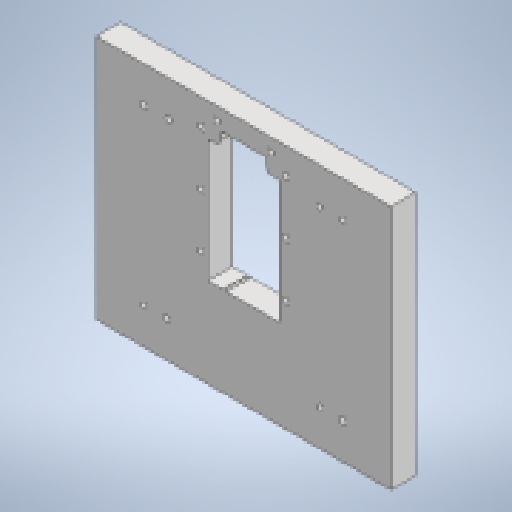
# Autodesk Inventor part: _body
Saved by Autodesk Inventor 2024.3 (Build 283343000, 343)
## iProperties
Created: 2024-09-06
Part Number: _body
Material: 일반
Document SubType Name: Modeling
Designer: gretc
Density: 1 g/cm^3
Appearance: 기본값
Author: gretc
Autodesk Inventor part; units mm, degrees
ref_plane "YZ Plane" through (0, 0, 0) normal (1, 0, 0) x (0, 1, 0)
ref_plane "XZ Plane" through (0, 0, 0) normal (0, 1, 0) x (-1, 0, 0)
ref_plane "XY Plane" through (0, 0, 0) normal (0, 0, 1) x (1, 0, 0)
ref_plane "작업 평면1" through (0, 0, 0) normal (0, 0, 1) x (1, 0, 0)
sketch "스케치1" plane through (0, 0, 0) normal (0, 0, 1) x (1, 0, 0)
  line L0 (-23.2, -18.48) -> (-93.2, -18.48) projected
  circle A0 centre (18.4, -3) radius 1.35 projected
  circle A1 centre (9.2, -3) radius 1.35 projected
  line L1 (0, 0) -> (27.6, 0) projected
  line L2 (0, 0) -> (0, -6) projected
  line L3 (0, -6) -> (27.6, -6) projected
  line L4 (27.6, 0) -> (27.6, -6) projected
  circle A2 centre (-62.8, -3) radius 1.35 projected
  circle A3 centre (-53.6, -3) radius 1.35 projected
  line L5 (-44.4, 0) -> (-72, 0) projected
  line L6 (-72, 0) -> (-72, -6) projected
  line L7 (-44.4, -6) -> (-72, -6) projected
  line L8 (-44.4, 0) -> (-44.4, -6) projected
  circle A4 centre (-62.8, 67.72) radius 1.35 projected
  circle A5 centre (-52.9755, 67.72) radius 1.35 projected
  line L9 (-44.4, 70.72) -> (-72, 70.72) projected
  line L10 (-72, 70.72) -> (-72, 64.72) projected
  line L11 (-44.4, 64.72) -> (-72, 64.72) projected
  line L12 (-44.4, 70.72) -> (-44.4, 64.72) projected
  circle A6 centre (18.4, 67.72) radius 1.35 projected
  circle A7 centre (8.5755, 67.72) radius 1.35 projected
  line L13 (0, 70.72) -> (27.6, 70.72) projected
  line L14 (0, 70.72) -> (0, 64.72) projected
  line L15 (0, 64.72) -> (27.6, 64.72) projected
  line L16 (27.6, 70.72) -> (27.6, 64.72) projected
  line L17 (0, 64.72) -> (-44.4, 64.72)
  line L18 (-44.4, 0) -> (-44.4, 64.72)
  line L19 (-22.2, 64.72) -> (-22.2, 32.36)
  line L20 (37.8, -17.64) -> (37.8, 82.36)
  line L21 (37.8, 82.36) -> (-82.2, 82.36)
  line L22 (-82.2, 82.36) -> (-82.2, -17.64)
  line L23 (-82.2, -17.64) -> (37.8, -17.64)
  line L24 (37.8, -17.64) -> (-82.2, 82.36) construction
  line L25 (37.8, 82.36) -> (-82.2, -17.64) construction
  dimension "d0" = 32.36
  dimension "d1" = 100
  dimension "d2" = 120
  constraints: 18 end point, 3 midpoint, 2 parallel, 2 perpendicular, 2 vertical, 1 collinear
  measures "d0" distance of L19.start L19.end
  measures "d1" distance of L20.start L20.end
  measures "d2" distance of L21.end L20.end
extrude "돌출1" add sketch "스케치1" along normal blind 10 contours L1 L4 L3 L2 | L8 L7 L6 L5 | L12 L11 L10 L9 | L13 L16 L15 L14 | L23 L22 L21 L20
sketch "스케치3" plane through (0, 0, 10) normal (0, 0, 1) x (1, 0, 0)
  arc A0 (-42.3, 27.1781) -> (-41.7808, 25.4912) centre (-39.3, 27.1781) ccw projected
  line L0 (-41.7808, 25.4912) -> (-37.7953, 19.6301) projected
  arc A1 (-37.7953, 19.6301) -> (-36.1414, 18.7547) centre (-36.1414, 20.7547) ccw projected
  line L1 (-35.2, 18.7547) -> (-36.1414, 18.7547) projected
  arc A2 (-36.7, 20.2547) -> (-35.2, 18.7547) centre (-35.2, 20.2547) ccw projected
  line L2 (-36.7, 73.2547) -> (-36.7, 20.2547) projected
  arc A3 (-35.7, 74.2547) -> (-36.7, 73.2547) centre (-35.7, 73.2547) ccw projected
  line L3 (-8.7, 74.2547) -> (-35.7, 74.2547) projected
  arc A4 (-7.7, 73.2547) -> (-8.7, 74.2547) centre (-8.7, 73.2547) ccw projected
  line L4 (-7.7, 20.2547) -> (-7.7, 73.2547) projected
  arc A5 (-9.2, 18.7547) -> (-7.7, 20.2547) centre (-9.2, 20.2547) ccw projected
  line L5 (-8.2586, 18.7547) -> (-9.2, 18.7547) projected
  arc A6 (-8.2586, 18.7547) -> (-6.6047, 19.6301) centre (-8.2586, 20.7547) ccw projected
  line L6 (-6.6047, 19.6301) -> (-2.6192, 25.4912) projected
  arc A7 (-2.6192, 25.4912) -> (-2.1, 27.1781) centre (-5.1, 27.1781) ccw projected
  line L7 (-2.1, 27.1781) -> (-2.1, 71.4314) projected
  arc A8 (-2.1, 71.4314) -> (-2.6192, 73.1183) centre (-5.1, 71.4314) ccw projected
  line L8 (-2.6192, 73.1183) -> (-6.3071, 78.5417) projected
  arc A9 (-6.3071, 78.5417) -> (-8.7879, 79.8547) centre (-8.7879, 76.8547) ccw projected
  line L9 (-8.7879, 79.8547) -> (-35.6121, 79.8547) projected
  arc A10 (-35.6121, 79.8547) -> (-38.0929, 78.5417) centre (-35.6121, 76.8547) ccw projected
  line L10 (-38.0929, 78.5417) -> (-41.7808, 73.1183) projected
  arc A11 (-41.7808, 73.1183) -> (-42.3, 71.4314) centre (-39.3, 71.4314) ccw projected
  line L11 (-42.3, 71.4314) -> (-42.3, 27.1781) projected
  circle A12 centre (-4.9, 27.7547) radius 1.35 projected
  circle A13 centre (-4.9, 49.7547) radius 1.35 projected
  circle A14 centre (-11.2, 77.0547) radius 1.35 projected
  circle A15 centre (-39.5, 27.7547) radius 1.35 projected
  circle A16 centre (-39.5, 49.7547) radius 1.35 projected
  circle A17 centre (-33.2, 77.0547) radius 1.35 projected
  circle A18 centre (-4.9, 71.7547) radius 1.35 projected
  circle A19 centre (-39.5, 71.7547) radius 1.35 projected
  point P0 (0, 0)
extrude "돌출2" cut sketch "스케치3" against normal blind 10 contours A12 | A13 | A14 | A15 | A16 | A17 | A18 | A19
sketch "스케치4" plane through (0, 0, 10) normal (0, 0, 1) x (1, 0, 0)
  circle A0 centre (-22.2, 31.7547) radius 7.5 projected
  circle A1 centre (-22.2, 31.7547) radius 7.5 projected
  point P0 (0, 0)
extrude "돌출3" cut sketch "스케치4" against normal blind 10
sketch "스케치5" plane through (0, 0, 10) normal (0, 0, 1) x (1, 0, 0)
  arc A0 (-42.3, 27.1781) -> (-41.7808, 25.4912) centre (-39.3, 27.1781) ccw projected
  line L0 (-42.3, 71.4314) -> (-42.3, 27.1781) projected
  arc A1 (-41.7808, 73.1183) -> (-42.3, 71.4314) centre (-39.3, 71.4314) ccw projected
  line L1 (-38.0929, 78.5417) -> (-41.7808, 73.1183) projected
  arc A2 (-35.6121, 79.8547) -> (-38.0929, 78.5417) centre (-35.6121, 76.8547) ccw projected
  line L2 (-8.7879, 79.8547) -> (-35.6121, 79.8547) projected
  arc A3 (-6.3071, 78.5417) -> (-8.7879, 79.8547) centre (-8.7879, 76.8547) ccw projected
  line L3 (-2.6192, 73.1183) -> (-6.3071, 78.5417) projected
  arc A4 (-2.1, 71.4314) -> (-2.6192, 73.1183) centre (-5.1, 71.4314) ccw projected
  line L4 (-2.1, 27.1781) -> (-2.1, 71.4314) projected
  arc A5 (-2.6192, 25.4912) -> (-2.1, 27.1781) centre (-5.1, 27.1781) ccw projected
  line L5 (-6.6047, 19.6301) -> (-2.6192, 25.4912) projected
  arc A6 (-8.2586, 18.7547) -> (-6.6047, 19.6301) centre (-8.2586, 20.7547) ccw projected
  line L6 (-14.55, 18.7547) -> (-8.2586, 18.7547) projected
  arc A7 (-14.55, 18.7547) -> (-13.05, 20.2547) centre (-14.55, 20.2547) ccw projected
  line L7 (-13.05, 20.2547) -> (-13.05, 21.7547) projected
  arc A8 (-10.7, 24.1047) -> (-13.05, 21.7547) centre (-10.7, 21.7547) ccw projected
  line L8 (-10.7, 24.1047) -> (-8.7, 24.1047) projected
  arc A9 (-8.7, 24.1047) -> (-7.7, 25.1047) centre (-8.7, 25.1047) ccw projected
  line L9 (-7.7, 25.1047) -> (-7.7, 67.9047) projected
  arc A10 (-7.7, 67.9047) -> (-8.7, 68.9047) centre (-8.7, 67.9047) ccw projected
  line L10 (-8.7, 68.9047) -> (-10.7, 68.9047) projected
  arc A11 (-13.05, 71.2547) -> (-10.7, 68.9047) centre (-10.7, 71.2547) ccw projected
  line L11 (-13.05, 71.2547) -> (-13.05, 73.2547) projected
  arc A12 (-13.05, 73.2547) -> (-14.05, 74.2547) centre (-14.05, 73.2547) ccw projected
  line L12 (-14.05, 74.2547) -> (-30.35, 74.2547) projected
  arc A13 (-30.35, 74.2547) -> (-31.35, 73.2547) centre (-30.35, 73.2547) ccw projected
  line L13 (-31.35, 73.2547) -> (-31.35, 71.2547) projected
  arc A14 (-33.7, 68.9047) -> (-31.35, 71.2547) centre (-33.7, 71.2547) ccw projected
  line L14 (-33.7, 68.9047) -> (-35.7, 68.9047) projected
  arc A15 (-35.7, 68.9047) -> (-36.7, 67.9047) centre (-35.7, 67.9047) ccw projected
  line L15 (-36.7, 67.9047) -> (-36.7, 25.1047) projected
  arc A16 (-36.7, 25.1047) -> (-35.7, 24.1047) centre (-35.7, 25.1047) ccw projected
  line L16 (-35.7, 24.1047) -> (-33.7, 24.1047) projected
  arc A17 (-31.35, 21.7547) -> (-33.7, 24.1047) centre (-33.7, 21.7547) ccw projected
  line L17 (-31.35, 21.7547) -> (-31.35, 20.2547) projected
  arc A18 (-31.35, 20.2547) -> (-29.85, 18.7547) centre (-29.85, 20.2547) ccw projected
  line L18 (-36.1414, 18.7547) -> (-29.85, 18.7547) projected
  arc A19 (-37.7953, 19.6301) -> (-36.1414, 18.7547) centre (-36.1414, 20.7547) ccw projected
  line L19 (-41.7808, 25.4912) -> (-37.7953, 19.6301) projected
  circle A20 centre (-4.9, 27.7547) radius 1.35 projected
  circle A21 centre (-4.9, 49.7547) radius 1.35 projected
  circle A22 centre (-11.2, 77.0547) radius 1.35 projected
  circle A23 centre (-39.5, 27.7547) radius 1.35 projected
  circle A24 centre (-39.5, 49.7547) radius 1.35 projected
  circle A25 centre (-33.2, 77.0547) radius 1.35 projected
  circle A26 centre (-4.9, 71.7547) radius 1.35 projected
  circle A27 centre (-39.5, 71.7547) radius 1.35 projected
  line L20 (-7.6, 67.9047) -> (-7.6, 25.1047)
  arc A28 (-8.7, 24.0047) -> (-7.6, 25.1047) centre (-8.7, 25.1047) ccw
  line L21 (-8.7, 24.0047) -> (-10.7, 24.0047)
  arc A29 (-10.7, 24.0047) -> (-12.95, 21.7547) centre (-10.7, 21.7547) ccw
  line L22 (-12.95, 21.7547) -> (-12.95, 20.2547)
  arc A30 (-13.7754, 18.8547) -> (-12.95, 20.2547) centre (-14.55, 20.2547) ccw
  line L23 (-13.7754, 18.8547) -> (-8.2586, 18.8547)
  arc A31 (-8.2586, 18.8547) -> (-6.6874, 19.6863) centre (-8.2586, 20.7547) ccw
  line L24 (-6.6874, 19.6863) -> (-2.7019, 25.5474)
  arc A32 (-2.7019, 25.5474) -> (-2.2, 27.1781) centre (-5.1, 27.1781) ccw
  line L25 (-2.2, 27.1781) -> (-2.2, 71.4314)
  arc A33 (-2.2, 71.4314) -> (-2.7019, 73.0621) centre (-5.1, 71.4314) ccw
  line L26 (-2.7019, 73.0621) -> (-6.3898, 78.4854)
  arc A34 (-6.3898, 78.4854) -> (-8.7879, 79.7547) centre (-8.7879, 76.8547) ccw
  line L27 (-8.7879, 79.7547) -> (-35.6121, 79.7547)
  arc A35 (-35.6121, 79.7547) -> (-38.0102, 78.4854) centre (-35.6121, 76.8547) ccw
  line L28 (-38.0102, 78.4854) -> (-41.6981, 73.0621)
  arc A36 (-41.6981, 73.0621) -> (-42.2, 71.4314) centre (-39.3, 71.4314) ccw
  line L29 (-42.2, 71.4314) -> (-42.2, 27.1781)
  arc A37 (-42.2, 27.1781) -> (-41.6981, 25.5474) centre (-39.3, 27.1781) ccw
  line L30 (-41.6981, 25.5474) -> (-37.7126, 19.6863)
  arc A38 (-37.7126, 19.6863) -> (-36.1414, 18.8547) centre (-36.1414, 20.7547) ccw
  line L31 (-36.1414, 18.8547) -> (-29.0754, 18.8547)
  arc A39 (-31.45, 20.2547) -> (-29.0754, 18.8547) centre (-29.85, 20.2547) ccw
  line L32 (-31.45, 20.2547) -> (-31.45, 21.7547)
  arc A40 (-31.45, 21.7547) -> (-33.7, 24.0047) centre (-33.7, 21.7547) ccw
  line L33 (-33.7, 24.0047) -> (-35.7, 24.0047)
  arc A41 (-36.8, 25.1047) -> (-35.7, 24.0047) centre (-35.7, 25.1047) ccw
  line L34 (-36.8, 25.1047) -> (-36.8, 67.9047)
  arc A42 (-35.7, 69.0047) -> (-36.8, 67.9047) centre (-35.7, 67.9047) ccw
  line L35 (-35.7, 69.0047) -> (-33.7, 69.0047)
  arc A43 (-33.7, 69.0047) -> (-31.45, 71.2547) centre (-33.7, 71.2547) ccw
  line L36 (-31.45, 71.2547) -> (-31.45, 73.2547)
  arc A44 (-30.35, 74.3547) -> (-31.45, 73.2547) centre (-30.35, 73.2547) ccw
  line L37 (-30.35, 74.3547) -> (-14.05, 74.3547)
  arc A45 (-12.95, 73.2547) -> (-14.05, 74.3547) centre (-14.05, 73.2547) ccw
  line L38 (-12.95, 73.2547) -> (-12.95, 71.2547)
  arc A46 (-12.95, 71.2547) -> (-10.7, 69.0047) centre (-10.7, 71.2547) ccw
  line L39 (-10.7, 69.0047) -> (-8.7, 69.0047)
  arc A47 (-7.6, 67.9047) -> (-8.7, 69.0047) centre (-8.7, 67.9047) ccw
  line L40 (-7.6, 25.1047) -> (-36.8, 25.1047)
  line L41 (-36.8, 25.1047) -> (-36.8, 18.7547)
  line L42 (-36.8, 18.7547) -> (-7.6, 18.7547)
  line L43 (-7.6, 18.7547) -> (-7.6, 25.1047)
  point P0 (0, 0)
  point P1 (-30.4068, 18.7547)
  point P2 (-30.3885, 18.8547)
  point P3 (-29.2932, 18.7547)
  point P4 (-8.2586, 18.7547)
  point P5 (-30.6246, 18.8547)
  dimension "d9" = 0.1
  constraints: 48 end point, 40 point on circle, 20 centre point, 2 parallel, 1 perpendicular, 39 other
  measures "d9" distance between parallel lines of L9 L20
extrude "돌출4" cut sketch "스케치5" against normal through all contours L41 A38 L31 A39 L18 A19 | A19 L42 L41 | L41 A41 L33 A40 L32 A39 L31 A38 | L40 A16 L16 A17 L17 A18 L31 A39 L32 A40 L33 A41 | L34 A42 L35 A43 L36 A44 L37 A45 L38 A46 L39 A47 L20 L40 L9 A10 L10 A11 L11 A12 L12 A13 L13 A14 L14 A15 L15 | A39 L31 A18 L17 A17 L16 A16 L40 A9 L8 A8 L7 A7 L42 | L15 A15 L14 A14 L13 A13 L12 A12 L11 A11 L10 A10 L9 L40 | A7 L7 A8 L8 A9 L40 A28 L21 A29 L22 A30 L23 A31 L43 A6 L6 | A6 L43 L42 | L43 A31 L23 A30 L22 A29 L21 A28
